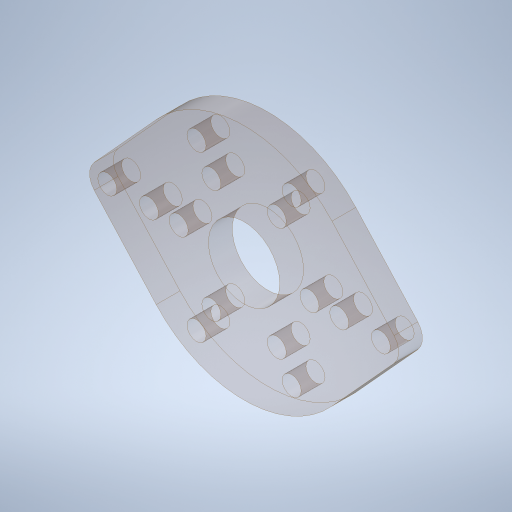
# Autodesk Inventor part: GP9-003
Saved by Autodesk Inventor 2023.4 (Build 274418000, 418)
## iProperties
Created: 2025-02-24
Part Number: GP9-003
Material: Polycarbonate, Smoke
Document SubType Name: Modeling
Designer: dlangdon
Density: 1.2 g/cm^3
Appearance: Polycarbonate - Smoked
Author: dlangdon
Autodesk Inventor part; units mm, degrees
ref_plane "YZ Plane" through (0, 0, 0) normal (1, 0, 0) x (0, 1, 0)
ref_plane "XZ Plane" through (0, 0, 0) normal (0, 1, 0) x (-1, 0, 0)
ref_plane "XY Plane" through (0, 0, 0) normal (0, 0, 1) x (1, 0, 0)
sketch "Sketch1" plane through (0, 0, 0) normal (0, 0, 1) x (1, 0, 0)
  circle A0 centre (0, 0) radius 9.525
  circle A1 centre (0, 0) radius 31.75 construction
  circle A2 centre (-36.5125, 0) radius 4.7625 construction
  circle A3 centre (36.5125, 0) radius 4.7625 construction
  circle A4 centre (0, 0) radius 17.4625 construction
  line L0 (-23.4674, 21.3856) -> (-40.0326, 3.2078)
  line L1 (-40.0326, -3.2078) -> (-23.4674, -21.3856)
  line L2 (23.4674, -21.3856) -> (40.0326, -3.2078)
  line L3 (40.0326, 3.2078) -> (23.4674, 21.3856)
  arc A5 (-40.0326, 3.2078) -> (-40.0326, -3.2078) centre (-36.5125, 0) ccw
  arc A6 (-23.4674, -21.3856) -> (23.4674, -21.3856) centre (0, 0) ccw
  arc A7 (40.0326, -3.2078) -> (40.0326, 3.2078) centre (36.5125, 0) ccw
  arc A8 (23.4674, 21.3856) -> (-23.4674, 21.3856) centre (0, 0) ccw
  line L4 (-36.5125, 0) -> (36.5125, 0) construction
  circle A9 centre (0, 0) radius 25.4 construction
  point P0 (-17.4625, 0)
  point P1 (-33.4211, -3.4732)
  point P2 (-25.4, 0)
  point P3 (-12.7, -21.997)
  point P4 (-8.7313, -15.123)
  point P5 (12.7, -21.997)
  point P6 (8.7312, -15.123)
  point P7 (25.4, 0)
  point P8 (17.4625, 0)
  point P9 (12.7, 21.997)
  point P10 (8.7313, 15.123)
  point P11 (-12.7, 21.997)
  point P12 (-8.7312, 15.123)
  dimension "d3" = 34.925
  dimension "d18" = 50.8
  dimension "d0" = 19.05
  dimension "d1" = 63.5
  dimension "d2" = 9.525
  dimension "d21" = 360
  constraints: 16 point on circle, 11 coincident, 10 end point, 9 tangent, 8 centre point, 5 horizontal alignment, 2 equal radius, 1 horizontal, 1 midpoint, 1 point on line, 17 other
  measures "d0" diameter of A0
  measures "d1" diameter of A1
  measures "d2" diameter of A2
extrude "Extrusion1" add sketch "Sketch1" along normal blind 6.35
hole "Hole2" at (-17.4625, 0, 0) at (-36.5125, 0, 0) at (36.5125, 0, 0) at (-25.4, 0, 0) at (-12.7, -21.997, 0) at (-8.7313, -15.123, 0) at (12.7, -21.997, 0) at (8.7312, -15.123, 0) at (25.4, 0, 0) at (17.4625, 0, 0) at (12.7, 21.997, 0) at (8.7313, 15.123, 0) at (-12.7, 21.997, 0) at (-8.7312, 15.123, 0) direction (0, 0, 1) diameter 5.1054 end through all clearance for "Flat Head Machine Screw (82)" size "#10" standard "Ansi Unified Screw Threads"
body "Solid1"
